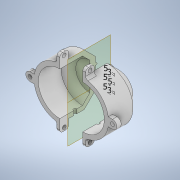
# Autodesk Inventor part: AirFeed1
Saved by Autodesk Inventor 2020.1 (Build 241239000, 239)
## iProperties
Created: 2019-11-11
Part Number: AirFeed1
Material: Generic
Document SubType Name: Modeling
Designer: Paul Lefeuvre
Density: 1 g/cm^3
Appearance: Default
Author: Paul Lefeuvre
Autodesk Inventor part; units mm, degrees
ref_plane "YZ Plane" through (0, 0, 0) normal (1, 0, 0) x (0, 1, 0)
ref_plane "XZ Plane" through (0, 0, 0) normal (0, 1, 0) x (-1, 0, 0)
ref_plane "XY Plane" through (0, 0, 0) normal (0, 0, 1) x (1, 0, 0)
sketch "Sketch1" plane through (0, 0, 0) normal (1, 0, 0) x (0, 1, 0)
  line L0 (37.4, 19.7) -> (37.4, -19.7)
  line L1 (37.4, -19.7) -> (-37.4, -19.7)
  line L2 (-37.4, -19.7) -> (-37.4, 19.7)
  line L3 (-37.4, 19.7) -> (37.4, -19.7) construction
  line L4 (37.4, 19.7) -> (-37.4, -19.7) construction
  line L5 (44.9, -22.6981) -> (44.9, 19.7)
  line L6 (-44.9, 19.7) -> (-44.9, -22.6981)
  line L7 (-44.9, -22.6981) -> (-25, -42.5981)
  line L8 (25, -42.5981) -> (44.9, -22.6981)
  line L9 (0, -42.5981) -> (0, -19.7) construction
  line L10 (-2.5, -19.7) -> (-2.5, -42.5981)
  line L11 (2.5, -19.7) -> (2.5, -42.5981)
  line L12 (37.4, 19.7) -> (44.9, 19.7)
  line L13 (-37.4, 19.7) -> (-44.9, 19.7)
  line L14 (25, -42.5981) -> (-25, -42.5981)
  line L15 (37.4, -19.7) -> (24.5019, -32.5981)
  line L16 (24.5019, -32.5981) -> (-24.5019, -32.5981)
  line L17 (-24.5019, -32.5981) -> (-37.4, -19.7)
  line L18 (-37.4, -9.7) -> (-44.9, -9.7)
  line L19 (-37.4, -4.2) -> (-44.9, -4.2)
  line L20 (-16.25, -42.5981) -> (-14.133, -45.1211)
  line L21 (-13.367, -45.1211) -> (-11.25, -42.5981)
  line L22 (-13.75, -45.5775) -> (-13.75, -42.5981)
  arc A0 (-14.133, -45.1211) -> (-13.367, -45.1211) centre (-13.75, -44.7997) ccw
  line L23 (-44.9, -4.2) -> (-48.8679, -4.2)
  line L24 (-48.8679, -4.2) -> (-48.8679, -9.7)
  line L25 (-48.8679, -9.7) -> (-44.9, -9.7)
  line L26 (-44.9, -9.7) -> (-44.9, -4.2)
  line L27 (-37.4, -9.7) -> (-35.2773, -9.7)
  line L28 (-35.2773, -9.7) -> (-35.2773, -4.2)
  line L29 (-35.2773, -4.2) -> (-37.4, -4.2)
  line L30 (-37.4, -4.2) -> (-37.4, -9.7)
  line L31 (-48.8679, -6.95) -> (-35.2773, -6.95)
  point P0 (0, 0)
  point P1 (2.5, -32.5981)
  point P2 (-2.5, -32.5981)
  point P3 (-13.75, -45.2997)
  point P4 (-37.4, -4.2)
  dimension "d0" = 74.8
  dimension "d2" = 7.5
  dimension "d3" = 45
  dimension "d4" = 45
  dimension "d5" = 7.5
  dimension "d7" = 2.5
  dimension "d8" = 2.5
  dimension "d9" = 50
  dimension "d22" = 10
  dimension "d23" = 5.5
  dimension "d24" = 10
  dimension "d30" = 8.75
  dimension "d31" = 8.75
  dimension "d32" = 40
  dimension "d33" = 40
  dimension "d34" = 0.5
  constraints: 63 end point, 9 parallel, 9 point on line, 7 perpendicular, 5 midpoint, 3 horizontal, 2 point on circle, 2 tangent, 2 vertical, 1 centre point, 10 other
  measures "d0" distance of L0.end L1.end
  measures "d2" distance between parallel lines of L0 L5
  measures "d3" angle of L1 L8
  measures "d4" angle of L1 L7
  measures "d5" distance between parallel lines of L2 L6
  measures "d7" distance between parallel lines of L11 L9
  measures "d8" distance between parallel lines of L9 L10
  measures "d9" distance of L7.end L8.start
  measures "d23" distance between parallel lines of L18 L19
  measures "d24" distance of L18.start L1.end
  measures "d30" distance of L7.end L20.start
  measures "d31" distance of L10.end L21.end
  measures "d32" angle of L21 L22
  measures "d33" angle of L22 L20
  measures "d34" radius of A0
revolve "Revolution1" add sketch "Sketch1" angle 360 about axis through (0, 0, -42.5981) along (0, 0, 1) contours L12 L5 L8 L14 L11 L16 L15 L0 | L17 L16 L10 L14 L7 L6 L18 L2 | L18 L6 L31 L2 | L31 L6 L19 L2 | L19 L6 L13 L2
revolve "Revolution2" add sketch "Sketch1" angle 360 about axis through (0, -13.75, -45.5775) along (0, 0, 1) contours L21 A0 L22 L14
revolve "Revolution3" cut sketch "Sketch1" angle 360 about axis through (0, -48.8679, -6.95) along (0, 1, 0) contours L31 L6 L19 L2 | L2 L29 L28 L31 | L31 L24 L23 L6
sketch "Sketch2" plane through (0, 0, 19.7) normal (0, 0, 1) x (1, 0, 0)
  arc A0 (0, 44.9) -> (0, -44.9) centre (0, 0) ccw projected
  line L0 (-44.2692, -7.5) -> (-44.2692, 7.5)
  line L1 (-44.2692, 7.5) -> (-51.7692, 7.5)
  line L2 (-59.2692, 0) -> (-59.2692, 0)
  line L3 (-51.7692, -7.5) -> (-44.2692, -7.5)
  arc A1 (0, -44.9) -> (0, 44.9) centre (0, 0) ccw projected
  arc A2 (0, 44.9) -> (0, -44.9) centre (0, 0) ccw projected
  circle A3 centre (-51.7692, 0) radius 3.3
  line L4 (-59.2692, 7.5) -> (-44.2692, -7.5) construction
  line L5 (-59.2692, -7.5) -> (-44.2692, 7.5) construction
  line L6 (-5, 44.6207) -> (5, 44.6207)
  line L7 (5, 44.6207) -> (5, 59.6207)
  line L8 (5, 59.6207) -> (-5, 59.6207)
  line L9 (-5, 59.6207) -> (-5, 44.6207)
  arc A4 (-51.7692, 7.5) -> (-59.2692, 0) centre (-51.7692, 0) ccw
  arc A5 (-59.2692, 0) -> (-51.7692, -7.5) centre (-51.7692, 0) ccw
  arc A6 (-8.998, 43.9892) -> (-5, 48.8877) centre (-10, 48.8877) ccw
  point P0 (0, 0)
  point P1 (-59.2692, 0)
  point P2 (-44.2692, 7.5)
  point P3 (-8.998, 43.9892)
  dimension "d37" = 15
  dimension "d38" = 15
  dimension "d39" = 6.6
  dimension "d40" = 10
  dimension "d41" = 15
  dimension "d42" = 7.5
  dimension "d43" = 5
  constraints: 20 end point, 12 point on circle, 6 tangent, 5 point on line, 4 centre point, 4 parallel, 2 horizontal, 2 perpendicular, 1 coincident, 1 concentric, 1 midpoint
  measures "d37" distance of L4.start L5.start
  measures "d38" distance of L0.end L4.start
  measures "d39" diameter of A3
  measures "d40" distance of L7.end L8.end
  measures "d41" distance of L6.end L7.end
  measures "d42" radius of A4
  measures "d43" radius of A6
extrude "Extrusion1" add sketch "Sketch2" against normal blind 7.5 contours A0 L3 A5 A4 L1
extrude "Extrusion2" add sketch "Sketch2" against normal blind 15 contours A0 L9 L8 L7 A1 | A0 A6 L9
ref_plane "Work Plane1" through (0, 37.4, 19.7) normal (-1, 0, 0) x (0, 1, 0)
mirror "Mirror1" about plane through (0, 37.4, 19.7) normal (-1, 0, 0) of "Extrusion2"
sketch "Sketch3" plane through (-5, 48.8877, 19.7) normal (-1, 0, 0) x (0, 0, 1)
  line L0 (-15, -4.8986) -> (-15, 0) projected
  line L1 (0, -4.267) -> (0, 10.733) projected
  line L2 (-15, 0) -> (0, 10.733) construction
  line L3 (-15, 0) -> (-15, 10.733) projected
  line L4 (0, 0) -> (0, -4.8986) projected
  line L5 (-15, 10.733) -> (0, 0) construction
  circle A0 centre (-7.5, 5.3665) radius 3.3
  line L6 (-13.4982, 1.0746) -> (-1.4997, 9.6599) construction
  line L7 (-1.5, 1.0756) -> (-13.5, 9.6574) construction
  circle A1 centre (-7.5, 5.3665) radius 4.9
  line L8 (0, 10.733) -> (-15, 10.733) projected
  arc A2 (-10, 10.733) -> (-15, 5.733) centre (-10, 5.733) ccw
  line L9 (0, 10.733) -> (-15, 10.733) projected
  arc A3 (0, 5.733) -> (-5, 10.733) centre (-5, 5.733) ccw
  line L10 (0, 10.733) -> (0, 0) projected
  point P0 (-19.7, -48.8877)
  point P1 (-5, 10.733)
  dimension "d48" = 6.6
  dimension "d51" = 9.8
  dimension "d52" = 5
  dimension "d53" = 5
  constraints: 8 end point, 6 point on line, 4 centre point, 4 point on circle, 4 tangent, 2 midpoint, 1 coincident
  measures "d48" diameter of A0
  measures "d51" diameter of A1
  measures "d52" radius of A2
  measures "d53" radius of A3
extrude "Extrusion3" cut sketch "Sketch3" against normal blind 10 contours A3 L8 L1 | L3 L8 A2 | A0
pattern_circular "Circular Pattern2" count 2 over 360 about axis through (0, 0, 0) along (0, 0, -1) of "Extrusion2", "Extrusion3", "Mirror1", "Extrusion1"
pattern_circular "Circular Pattern3" count 6 over 360 about axis through (0, 0, 0) along (0, 0, -1) of "Revolution2"
split body "Split1" result two bodies by plane through (0, 37.4, 19.7) normal (-1, 0, 0) first body at (-40.8617, -17.369, -8.5654)
sketch "Sketch5" plane through (0, 0, -42.5981) normal (0, 0, -1) x (-1, 0, 0)
  line L0 (0, 13.75) -> (0, 13.367) projected
  circle A0 centre (0, 13.75) radius 2.5
  line L1 (0, -13.367) -> (0, -13.75) projected
  circle A1 centre (0, -13.75) radius 2.5
  circle A2 centre (0, 13.75) radius 5.5
  circle A3 centre (0, -13.75) radius 5.5
  circle A4 centre (0, 0) radius 2.5
  circle A5 centre (0, 0) radius 7.5
  arc A6 (4.9453, 8.1114) -> (-4.9453, 8.1114) centre (0, 13.75) ccw
  arc A7 (4.9453, -8.1114) -> (4.9453, 8.1114) centre (0, 0) ccw
  arc A8 (-4.9453, -8.1114) -> (4.9453, -8.1114) centre (0, -13.75) ccw
  arc A9 (-4.9453, 8.1114) -> (-4.9453, -8.1114) centre (0, 0) ccw
  dimension "d69" = 3
  dimension "d70" = 3
  dimension "d71" = 5
  dimension "d72" = 5
  dimension "d73" = 5
  dimension "d74" = 5
  constraints: 10 centre point, 8 point on circle, 1 coincident
  measures "d69" radial gap between concentric circles of A0 A2
  measures "d70" radial gap between concentric circles of A1 A3
  measures "d71" radial gap between concentric circles of A4 A5
  measures "d72" diameter of A1
  measures "d73" diameter of A0
  measures "d74" diameter of A4
move or copy body "Move Body2" bodies to move or copy 2 copy no translate (-20, 0, 0)
move or copy body "Move Body3" bodies to move or copy 3 copy no translate (20, 0, 0)
extrude "Extrusion4" add sketch "Sketch5" along normal blind 7.5 contours A0 | A1 | A2 | A3 | A5 bodies 3
extrude "Extrusion5" add sketch "Sketch5" along normal blind 2.5 contours A0 | A1 | A2 | A3 | A5 | A7 A8 A9 A6 bodies 3
equation "\"d4\" = d3"
equation "\"d8\" = d7"
body "Solid2"
body "Solid3"
